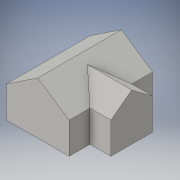
# Autodesk Inventor part: Figure 7_28_5
Saved by Autodesk Inventor 2016 (Build 200138000, 138)
## iProperties
Created: 2016-07-19
Part Number: Figure 7_28_5
Material: Generic
Document SubType Name: Modeling
Designer: cfkguest
Density: 1 g/cm^3
Appearance: Default
Author: cfkguest
Autodesk Inventor part; units mm, degrees
ref_plane "YZ Plane" through (0, 0, 0) normal (1, 0, 0) x (0, 1, 0)
ref_plane "XZ Plane" through (0, 0, 0) normal (0, 1, 0) x (-1, 0, 0)
ref_plane "XY Plane" through (0, 0, 0) normal (0, 0, 1) x (1, 0, 0)
sketch "Sketch1" plane through (0, 0, 0) normal (0, 0, 1) x (1, 0, 0)
  line L0 (-37.7472, -6.4088) -> (0.3528, -6.4088)
  line L1 (0.3528, -6.4088) -> (0.3528, 12.6412)
  line L2 (0.3528, 12.6412) -> (-18.6972, 25.3412)
  line L3 (-18.6972, 25.3412) -> (-37.7472, 12.6412)
  line L4 (-37.7472, 12.6412) -> (-37.7472, -6.4088)
  point P0 (0, 0)
  dimension "d0" = 19.05
  dimension "d1" = 19.05
  dimension "d2" = 38.1
  dimension "d3" = 12.7
  dimension "d4" = 19.05
  constraints: 10 end point, 1 horizontal, 1 parallel, 1 perpendicular
  measures "d0" distance of L3.end L0.start
  measures "d1" distance of L0.end L1.end
  measures "d2" distance of L0.start L0.end
  measures "d3" vertical distance of L3.end L2.end
  measures "d4" horizontal distance of L3.end L2.end
extrude "Extrusion1" add sketch "Sketch1" along normal blind 50.8
sketch "Sketch2" plane through (0.3528, -6.4088, 0) normal (1, 0, 0) x (0, 0, -1)
  line L0 (0, 19.05) -> (-50.8, 19.05) projected
  line L1 (-38.1, 19.05) -> (-38.1, 0)
  line L2 (0, 0) -> (-50.8, 0) projected
  line L3 (-38.1, 19.05) -> (-25.4, 28.575)
  line L4 (-25.4, 28.575) -> (-12.7, 19.05)
  line L5 (-12.7, 19.05) -> (-12.7, 0)
  line L6 (-12.7, 0) -> (-38.1, 0)
  line L7 (-50.8, 19.05) -> (-50.8, 0) projected
  line L8 (0, 0) -> (0, 19.05) projected
  point P0 (0, 6.4088)
  dimension "d7" = 12.7
  dimension "d8" = 12.7
  dimension "d9" = 9.525
  dimension "d10" = 12.7
  constraints: 10 end point, 4 point on line, 1 collinear, 1 parallel, 1 vertical
  measures "d7" distance between parallel lines of L7 L1
  measures "d8" distance between parallel lines of L8 L5
  measures "d9" vertical distance of L4.end L3.end
  measures "d10" horizontal distance of L3.end L4.end
extrude "Extrusion2" add sketch "Sketch2" along normal blind 12.7 and the other way blind 17.78 contours L5 L2 L1 L0 | L0 L3 L4
body "Solid1"
